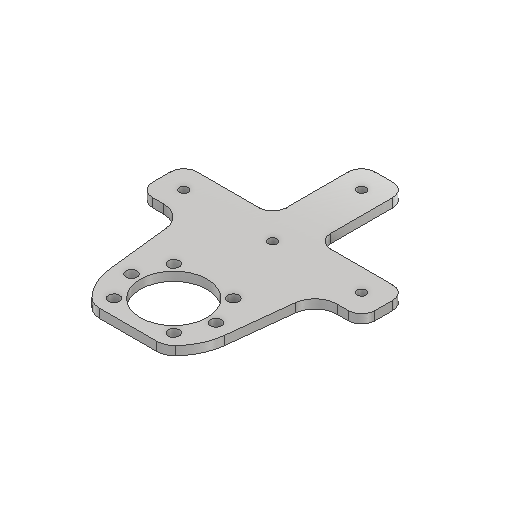
# Autodesk Inventor part: LC_ALU_4mm_Heatbed_Frame_Ball_Screw_Nut_Mounting_Bracket
Saved by Autodesk Inventor 2026.1 (Build 301233000, 233)
## iProperties
Created: 2016-06-21
Part Number: LC_ALU_4mm_Heatbed_Frame_Ball_Screw_Nut_Mounting_Bracket
Material: Ogólny
Document SubType Name: Modeling
Designer: Andrzej
Density: 1 g/cm^3
Appearance: Obrobione - aluminium
Mass: 19.2274 g
Surface Area: 120.946 cm^2
Volume: 19.2274 cm^3
Author: Andrzej
Autodesk Inventor part; units mm, degrees
ref_plane "YZ Plane" through (0, 0, 0) normal (1, 0, 0) x (0, 1, 0)
ref_plane "XZ Plane" through (0, 0, 0) normal (0, 1, 0) x (-1, 0, 0)
ref_plane "XY Plane" through (0, 0, 0) normal (0, 0, 1) x (1, 0, 0)
sketch "Szkic1" plane through (0, 0, 0) normal (0, 0, 1) x (1, 0, 0)
  line L0 (-47.736, 26.7667) -> (-47.736, 6.7667)
  line L1 (-47.736, 26.7667) -> (52.264, 26.7667)
  line L2 (52.264, 26.7667) -> (52.264, 6.7667)
  line L3 (52.264, 6.7667) -> (32.264, 6.7667)
  line L4 (32.264, 6.7667) -> (32.264, -48.2333)
  line L5 (32.264, -48.2333) -> (-27.736, -48.2333)
  line L6 (-27.736, -48.2333) -> (-27.736, 6.7667)
  line L7 (-27.736, 6.7667) -> (-47.736, 6.7667)
  circle A0 centre (2.264, -27.7333) radius 19
  arc A1 (-11.0025, -7.7333) -> (-11.0025, -47.7333) centre (2.264, -27.7333) ccw
  line L8 (-11.0025, -47.7333) -> (15.5305, -47.7333)
  arc A2 (15.5305, -47.7333) -> (15.5305, -7.7333) centre (2.264, -27.7333) ccw
  line L9 (15.5305, -7.7333) -> (-11.0025, -7.7333)
  circle A3 centre (2.264, -27.7333) radius 15
  circle A4 centre (-37.736, 16.7667) radius 2
  circle A5 centre (2.264, 16.7667) radius 2
  circle A6 centre (42.264, 16.7667) radius 2
  arc A7 (-23.5765, -30.609) -> (-13.7282, -48.2333) centre (2.264, -27.7333) ccw
  arc A8 (18.2561, -48.2333) -> (28.1044, -30.609) centre (2.264, -27.7333) ccw
  line L10 (-27.736, 6.7667) -> (-23.5765, -30.609)
  line L11 (32.264, 6.7667) -> (28.1044, -30.609)
  line L12 (-7.736, 26.7667) -> (-7.736, 66.7667)
  line L13 (-7.736, 66.7667) -> (12.264, 66.7667)
  line L14 (12.264, 66.7667) -> (12.264, 26.7667)
  circle A9 centre (2.264, 56.7667) radius 2
  point P0 (0, 0)
  point P1 (-16.736, -27.7333)
  point P2 (-11.1711, -41.1683)
  point P3 (15.699, -14.2982)
  point P4 (15.699, -41.1683)
  point P5 (-11.1711, -14.2982)
  point P6 (21.264, -27.7333)
  dimension "d0" = 20
  dimension "d1" = 100
  dimension "d2" = 20
  dimension "d3" = 60
  dimension "d4" = 20
  dimension "d5" = 55
  dimension "d8" = 38
  dimension "d13" = 34.5
  dimension "d14" = 30
  dimension "d15" = 30
  dimension "d24" = 4
  dimension "d25" = 4
  dimension "d26" = 4
  dimension "d29" = 10
  dimension "d30" = 10
  dimension "d31" = 10
  dimension "d32" = 10
  dimension "d33" = 10
  dimension "d34" = 50
  dimension "d42" = 2
  dimension "d47" = 40
  dimension "d48" = 20
  dimension "d49" = 40
  dimension "d50" = 10
  dimension "d51" = 10
  dimension "d52" = 4
  constraints: 30 end point, 13 point on circle, 10 centre point, 8 perpendicular, 5 point on line, 2 coincident, 2 tangent, 2 vertical, 1 horizontal
  measures "d0" distance of L0.start L0.end
  measures "d1" distance of L0.start L1.end
  measures "d2" distance of L2.end L3.end
  measures "d3" distance of L4.end L5.end
  measures "d4" distance of L6.end L0.end
  measures "d5" distance between parallel lines of L7 L5
  measures "d8" diameter of A0
  measures "d13" distance from line of point (2.264, -27.733) L7
  measures "d14" distance from line of L6 point (2.264, -27.733)
  measures "d15" diameter of A3
  measures "d24" diameter of A4
  measures "d25" diameter of A5
  measures "d26" diameter of A6
  measures "d29" distance from line of L0 A4.centre
  measures "d30" distance from line of L1 A4.centre
  measures "d31" distance from line of L1 A5.centre
  measures "d32" distance from line of L1 A6.centre
  measures "d33" distance from line of L2 A6.centre
  measures "d34" distance from line of L0 A5.centre
  measures "d42" radial gap between concentric circles of A1 A7
  measures "d47" distance of L12.start L12.end
  measures "d48" distance of L12.end L13.end
  measures "d49" distance between parallel lines of L0 L12
  measures "d50" distance from line of L12 point (2.264, 56.767)
  measures "d51" distance from line of point (2.264, 56.767) L13
  measures "d52" diameter of A9
extrude "Wyciągnięcie proste1" add sketch "Szkic1" along normal blind 4 contours L1 L2 L3 L11 A8 L5 A7 L10 L7 L0 | L12 L13 L14 L1 | L10 A7 L5 L6 | A8 L11 L4 L5 | A0 | L9 A2 L8 A1 | A3 | A4 | A5 | A6 | A9
extrude "Wyciągnięcie proste2" cut sketch "Szkic1" along normal through all contours A3 | A4 | A5 | A6 | A9
hole "Otwór1" at (2.264, -27.7333, 0) at (21.264, -27.7333, 0) at (-11.1711, -41.1683, 0) at (15.699, -41.1683, 0) at (15.699, -14.2982, 0) at (-11.1711, -14.2982, 0) at (-16.736, -27.7333, 0) direction (0, 0, 1) diameter 5 end through all
extrude "Wyciągnięcie proste3" cut sketch "Szkic1" along normal blind 10 contours L10 A7 L5 L6 | A8 L11 L4 L5
fillet "Zaokrąglenie1" radius 6 8 edges at (-47.736, 6.7667, 2) (-47.736, 26.7667, 2) (52.264, 6.7667, 2) (52.264, 26.7667, 2) (-7.736, 26.7667, 2) (-7.736, 66.7667, 2) (12.264, 26.7667, 2) (12.264, 66.7667, 2)
fillet "Zaokrąglenie2" radius 10 2 edges at (-27.736, 6.7667, 2) (32.264, 6.7667, 2)
fillet "Zaokrąglenie3" radius 8 2 edges at (-13.7282, -48.2333, 2) (18.2561, -48.2333, 2)
equation "\"d2\" = -0.5 * d3 + 0.5 * d1"
equation "\"d14\" = 0.5 * d3"
equation "\"d34\" = 0.5 * d1"
